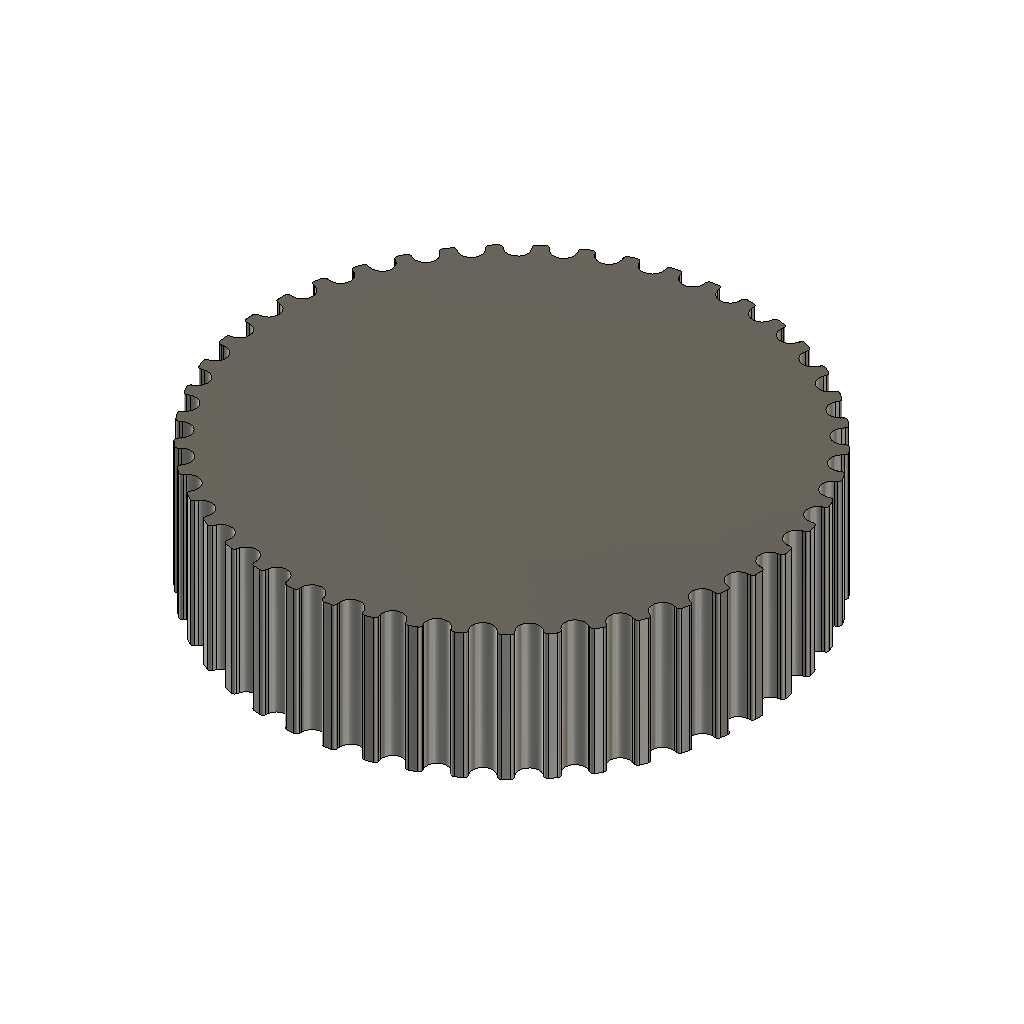
HTD-5M Generator (Autodesk Fusion 360 design; units mm, degrees)
Autodesk Fusion 360 part; units mm, degrees
sketch "Teeth" plane through (0, 0, 0) normal (0, 0, 1) x (1, 0, 0)
  circle A0 centre (0, 0) radius 35.8099
  arc A1 (0.4841, 35.2346) -> (0, 35.2379) centre (0, 0) ccw
  arc A2 (0.9071, 34.8346) -> (0.4841, 35.2346) centre (0.4782, 34.8046) ccw
  line L0 (0.9071, 34.8346) -> (0.9319, 34.4796)
  arc A3 (0.9319, 34.4796) -> (2.3144, 33.0971) centre (2.4183, 34.5834) ccw
  line L1 (0, 0) -> (0, 35.2379) construction
  line L2 (0, 0) -> (2.4183, 34.5834) construction
  line L3 (0, 35.2379) -> (0, 35.8099)
  arc A4 (2.498, 35.7227) -> (0, 35.8099) centre (0, 0) ccw
  arc A5 (2.3144, 33.0971) -> (3.8758, 34.2738) centre (2.4183, 34.5834) ccw
  line L4 (3.9497, 34.6218) -> (3.8758, 34.2738)
  arc A6 (4.4243, 34.959) -> (3.9497, 34.6218) centre (4.3703, 34.5324) ccw
  arc A7 (4.9042, 34.895) -> (4.4243, 34.959) centre (0, 0) ccw
  line L5 (4.9042, 34.895) -> (4.9838, 35.4614)
  arc A8 (4.9838, 35.4614) -> (2.498, 35.7227) centre (0, 0) ccw
  line L6 (0.9071, 34.8346) -> (2.4284, 34.7282) construction
  line L7 (2.4284, 34.7282) -> (2.4183, 34.5834) construction
  dimension "d50" = 71.6198
  dimension "d57" = 0.43
  dimension "d58" = 1.49
  dimension "d59" = 4
  dimension "d62" = 2.632
  dimension "d65" = 0.572
  dimension "d67" = 1.525
  constraint tangent A1 A2
  constraint coincident A0.centre A1.centre
  constraint vertical A0.centre A1.end
  constraint coincident A0 L3.end
  constraint parallel L1 L3
  constraint coincident A0 A4.start
  constraint collinear A3.centre A0.centre A4.start
  constraint coincident A3.centre L2.end
  constraint coincident L2 A3.end
  constraint symmetric L0.end L2 A5.end
  constraint symmetric A2.start L2 L4.start
  constraint symmetric A1.start L2 A6.start
  constraint symmetric A1 L2 A7
  constraint symmetric A2 L2 A6
  constraint symmetric A3 L2 A5
  constraint symmetric L2 A1.end A7.start
  constraint symmetric L2 L3.end L5.end
  constraint symmetric L2 A4.start A8.end
  constraint symmetric L2 A4 A8
  constraint symmetric L2 A3.end A5.start
  constraint tangent L0 A3
  constraint tangent A2 L0
  constraint perpendicular L2 L6
  constraint parallel L2 L7
  measures "d50" diameter of A0
  measures "d57" radius of A2
  measures "d58" radius of A3
  measures "d59" angle of L1 L2
  measures "d62" distance of A4.start A3.end
  measures "d65" distance of A1.end L3.end
  measures "d67" distance of A2.start L6.end
extrude "Extrude1" add sketch "Teeth" along normal mid plane 18.5
extrude "Extrude3" cut sketch "Teeth" along normal through all and the other way through all contours A0 A1 A2 L0 A3 L3 A4 A5 L4 A6 A7 L5 A8
pattern_circular "C-Pattern1" count 45 over 360 about axis through (0, 0, 0) along (0, 0, 1) of "Extrude3"
equation "p = 5 mm"
equation "n = 45" comment "Number of Teeth"
equation "PD = n * p / 3.14159"
equation "d25 = width"
equation "d50 = PD"
equation "d52 = n"
equation "d59 = ( 180 / n ) * 1 deg"
equation "width = 18.5 mm"
equation "d67 = 3.05 mm / 2"
